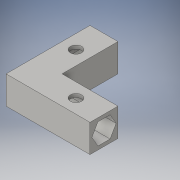
# Autodesk Inventor part: 3_8_angleJoint
Saved by Autodesk Inventor 2016 SP1 (Build 200210100, 210)
## iProperties
Created: 2015-11-23
Part Number: 3_8_angleJoint
Material: Generic
Document SubType Name: Modeling
Designer: steele
Density: 1 g/cm^3
Appearance: Default
Author: steele
Autodesk Inventor part; units mm, degrees
ref_plane "YZ Plane" through (0, 0, 0) normal (1, 0, 0) x (0, 1, 0)
ref_plane "XZ Plane" through (0, 0, 0) normal (0, 1, 0) x (-1, 0, 0)
ref_plane "XY Plane" through (0, 0, 0) normal (0, 0, 1) x (1, 0, 0)
sketch "Sketch1" plane through (0, 0, 0) normal (0, 1, 0) x (-1, 0, 0)
  line L0 (0, 0) -> (0, -25.4)
  line L1 (0, -25.4) -> (12.7, -25.4)
  line L2 (12.7, -25.4) -> (12.7, 12.7)
  line L3 (12.7, 12.7) -> (-25.4, 12.7)
  line L4 (-25.4, 12.7) -> (-25.4, 0)
  line L5 (-25.4, 0) -> (0, 0)
  dimension "d0" = 12.7
  dimension "d1" = 38.1
  constraints: 12 end point, 7 perpendicular, 1 vertical
  measures "d0" distance of L0.end L1.end
  measures "d1" distance of L1.end L2.end
extrude "Extrusion1" add sketch "Sketch1" against normal blind 12.7
sketch "Sketch3" plane through (0, 0, -25.4) normal (0, 0, -1) x (-1, 0, 0)
  line L0 (3.6004, -1.5875) -> (9.0996, -1.5875)
  line L1 (9.0996, -1.5875) -> (11.8493, -6.35)
  line L2 (11.8493, -6.35) -> (9.0996, -11.1125)
  line L3 (9.0996, -11.1125) -> (3.6004, -11.1125)
  line L4 (3.6004, -11.1125) -> (0.8507, -6.35)
  line L5 (0.8507, -6.35) -> (3.6004, -1.5875)
  line L6 (12.7, -12.7) -> (0, -12.7) projected
  line L7 (0, 0) -> (0, -12.7) projected
  point P0 (6.35, -6.35)
  dimension "d5" = 6.35
  dimension "d6" = 6.35
  dimension "d7" = 9.525
  constraints: 12 end point, 1 parallel, 13 other
  measures "d5" distance from line of L7 point (6.35, -6.35)
  measures "d6" distance from line of point (6.35, -6.35) L6
  measures "d7" distance between parallel lines of L0 L3
extrude "Extrusion2" cut sketch "Sketch3" against normal blind 31.75
sketch "Sketch4" plane through (25.4, 0, 12.7) normal (1, 0, 0) x (0, 0, -1)
  line L0 (11.8493, -6.35) -> (9.0996, -11.1125)
  line L1 (9.0996, -11.1125) -> (3.6004, -11.1125)
  line L2 (3.6004, -11.1125) -> (0.8507, -6.35)
  line L3 (0.8507, -6.35) -> (3.6004, -1.5875)
  line L4 (3.6004, -1.5875) -> (9.0996, -1.5875)
  line L5 (9.0996, -1.5875) -> (11.8493, -6.35)
  line L6 (0, 0) -> (12.7, 0) projected
  line L7 (12.7, 0) -> (12.7, -12.7) projected
  point P0 (6.35, -6.35)
  dimension "d10" = 9.525
  dimension "d11" = 6.35
  dimension "d12" = 6.35
  constraints: 12 end point, 1 parallel, 13 other
  measures "d10" distance between parallel lines of L1 L4
  measures "d11" distance from line of L7 point (6.35, -6.35)
  measures "d12" distance from line of point (6.35, -6.35) L6
extrude "Extrusion3" cut sketch "Sketch4" against normal blind 31.75
sketch "Sketch5" plane through (0, 0, 0) normal (0, 1, 0) x (1, 0, 0)
  line L0 (-12.7, 25.4) -> (-12.7, -12.7) projected
  line L1 (-12.7, -12.7) -> (25.4, -12.7) projected
  line L2 (0, 25.4) -> (-12.7, 25.4) projected
  line L3 (25.4, -12.7) -> (25.4, 0) projected
  point P0 (0, 0)
  point P1 (-6.35, 12.7)
  point P2 (12.7, -6.35)
  dimension "d15" = 6.35
  dimension "d16" = 6.35
  dimension "d17" = 12.7
  dimension "d18" = 12.7
  measures "d15" distance from line of point (-6.35, 12.7) L0
  measures "d16" distance from line of L1 point (12.7, -6.35)
  measures "d17" distance from line of point (-6.35, 12.7) L2
  measures "d18" distance from line of point (12.7, -6.35) L3
hole "Hole1" at (-6.35, 0, -12.7) at (12.7, 0, 6.35) direction (0, -1, 0) diameter 5.1054 end through all clearance for "Flat Head Machine Screw (82)" size "#10" standard "Ansi Unified Screw Threads"
equation "\"d0\" = pieceWidth"
equation "\"d1\" = pieceLength"
equation "\"d2\" = pieceWidth"
equation "\"d5\" = 0.5 * pieceWidth"
equation "\"d6\" = 0.5 * pieceWidth"
equation "\"d7\" = hex"
equation "\"d8\" = depthOfHexCut"
equation "\"d10\" = hex"
equation "\"d11\" = 0.5 * pieceWidth"
equation "\"d12\" = 0.5 * pieceWidth"
equation "\"d13\" = depthOfHexCut"
equation "\"d15\" = 0.5 * pieceWidth"
equation "\"d16\" = 0.5 * pieceWidth"
equation "\"d17\" = 0.5 * depthOfInsert"
equation "\"d18\" = 0.5 * depthOfInsert"
equation "\"hex\" = 9.525"
equation "\"pieceWidth\" = 12.7"
equation "\"pieceLength\" = 38.1"
equation "\"depthOfInsert\" = 25.4"
equation "\"depthOfHexCut\" = 31.75"
body "Solid1"
